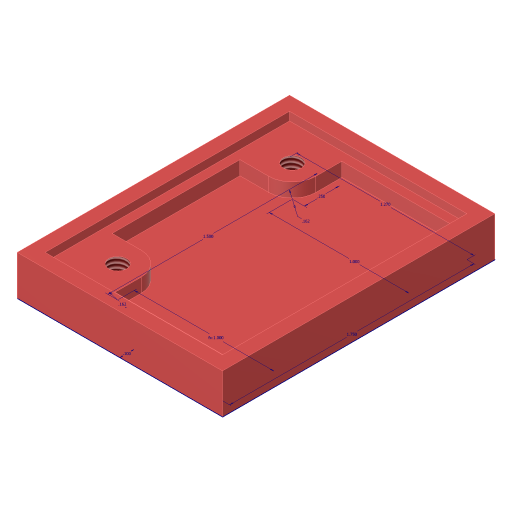
# Autodesk Inventor part: TOF mount
Saved by Autodesk Inventor 2023.4 (Build 274418000, 418)
## iProperties
Created: 2025-02-18
Part Number: TOF mount
Material: ABS Plastic
Document SubType Name: Modeling
Designer: mavericks
Density: 1.06 g/cm^3
Appearance: Smooth - Red
Author: mavericks
Autodesk Inventor part; units mm, degrees
ref_plane "YZ Plane" through (0, 0, 0) normal (1, 0, 0) x (0, 1, 0)
ref_plane "XZ Plane" through (0, 0, 0) normal (0, 1, 0) x (-1, 0, 0)
ref_plane "XY Plane" through (0, 0, 0) normal (0, 0, 1) x (1, 0, 0)
sketch "Sketch2" plane through (0, 0, 0) normal (0, 1, 0) x (-1, 0, 0)
  line L0 (16.129, 22.225) -> (-16.129, 22.225)
  line L1 (-16.129, 22.225) -> (-16.129, -22.225)
  line L2 (-16.129, -22.225) -> (16.129, -22.225)
  line L3 (16.129, -22.225) -> (16.129, 22.225)
  line L4 (16.129, 22.225) -> (-16.129, -22.225) construction
  line L5 (-16.129, 22.225) -> (16.129, -22.225) construction
  line L6 (-18.669, 24.765) -> (18.669, 24.765)
  line L7 (18.669, 24.765) -> (18.669, -24.765)
  line L8 (18.669, -24.765) -> (-18.669, -24.765)
  line L9 (-18.669, -24.765) -> (-18.669, 24.765)
  circle A0 centre (9.271, 15.875) radius 2.0574 construction
  circle A1 centre (9.271, -15.875) radius 2.0574 construction
  point P0 (0, 0)
  dimension "d0" = 32.258
  dimension "d1" = 44.45
  dimension "d2" = 2.54
  dimension "d32" = 25.4
  dimension "d33" = 25.4
  dimension "d34" = 6.35
  dimension "d35" = 38.1
  dimension "d43" = 4.1148
  dimension "d44" = 4.1148
  constraints: 20 end point, 4 parallel, 2 centre point, 2 coincident, 2 midpoint, 2 perpendicular, 1 horizontal, 3 other
  measures "d0" distance of L2.end L1.end
  measures "d1" distance of L1.end L0.end
  measures "d2" distance between parallel lines of L0 L6
  measures "d32" distance from line of L1 point (9.271, -15.875)
  measures "d33" distance from line of L1 point (9.271, 15.875)
  measures "d34" distance from line of point (9.271, -15.875) L2
  measures "d35" distance from line of point (9.271, 15.875) L2
  measures "d43" diameter of A0
  measures "d44" diameter of A1
extrude "Extrusion1" add sketch "Sketch2" along normal blind 3.175 contours L3 L2 L1 L0
extrude "Extrusion2" add sketch "Sketch2" along normal blind 7.239
sketch "Sketch5" plane through (0, 3.175, 0) normal (0, 1, 0) x (1, 0, 0)
  point P0 (0, 0)
sketch "Sketch6" plane through (0, 3.175, 0) normal (0, 1, 0) x (1, 0, 0)
  line L0 (16.129, -22.225) -> (16.129, 22.225) projected
  line L1 (16.129, -20.6375) -> (-14.5415, -20.6375)
  line L2 (-14.5415, -20.6375) -> (-14.5415, 20.6375)
  line L3 (-14.5415, 20.6375) -> (16.129, 20.6375)
  line L4 (-16.129, -22.225) -> (16.129, -22.225) projected
  line L5 (-16.129, 22.225) -> (-16.129, -22.225) projected
  line L6 (16.129, 22.225) -> (-16.129, 22.225) projected
  line L7 (16.129, -22.225) -> (16.129, 22.225) projected
  line L8 (16.129, 22.225) -> (-16.129, 22.225) projected
  line L9 (-16.129, 22.225) -> (-16.129, -22.225) projected
  line L10 (-16.129, -22.225) -> (16.129, -22.225) projected
  line L11 (-5.0165, -20.6375) -> (-5.0165, -15.875)
  line L12 (-9.271, -11.6205) -> (-14.5415, -11.6205)
  line L13 (-14.5415, 11.6205) -> (-9.271, 11.6205)
  line L14 (-5.0165, 15.875) -> (-5.0165, 20.6375)
  arc A0 (-5.0165, -15.875) -> (-9.271, -11.6205) centre (-9.271, -15.875) ccw
  arc A1 (-9.271, 11.6205) -> (-5.0165, 15.875) centre (-9.271, 15.875) ccw
  circle A2 centre (-9.271, -15.875) radius 2.0574 construction
  circle A3 centre (-9.271, 15.875) radius 2.0574 construction
  point P0 (0, 0)
  dimension "d23" = 1.5875
  dimension "d24" = 1.5875
  dimension "d25" = 1.5875
  dimension "d29" = 9.525
  dimension "d31" = 9.525
  constraints: 14 end point, 6 point on line, 4 perpendicular, 4 point on circle, 4 tangent, 2 centre point, 2 concentric, 2 horizontal, 1 vertical
  measures "d23" distance between parallel lines of L4 L1
  measures "d24" distance between parallel lines of L2 L5
  measures "d25" distance between parallel lines of L6 L3
  measures "d29" distance between parallel lines of L2 L11
  measures "d31" distance between parallel lines of L2 L14
extrude "Extrusion4" add sketch "Sketch6" along normal blind 2.54 contours L4 L5 L6 L0 L3 L2 L1 | L1 L2 L12 A0 L11 | L14 A1 L13 L2 L3
hole "Hole2" at (-9.271, 0, 15.875) at (-9.271, 0, -15.875) direction (0, 1, 0) diameter 3.302 end through all thread size "8-32 UNC" class "2B" standard "ANSI Unified Screw Threads"
equation "\"d33\" = d32"
equation "\"d31\" = d29"
body "Solid1"
